LCD_BUCK_MODULE (Autodesk Fusion 360 design; units mm, degrees)
Autodesk Fusion 360 part; units mm, degrees
sketch "Esquisse1" plane through (0, 0, 0) normal (0, 0, 1) x (1, 0, 0)
  line L0 (-36, -19) -> (36, -19)
  line L1 (36, -19) -> (36, 19)
  line L2 (36, 19) -> (-36, 19)
  line L3 (-36, 19) -> (-36, -19)
  line L4 (-36, -19) -> (36, 19) construction
  line L5 (36, -19) -> (-36, 19) construction
  line L6 (-36, -6.0464) -> (-38, -6.0464)
  line L7 (-38, -6.0464) -> (-38, 5.9536)
  line L8 (-38, 5.9536) -> (-36, 5.9536)
  line L9 (-36, 5.9536) -> (-36, -6.0464)
  line L10 (-36, -6.0464) -> (-38, 5.9536) construction
  line L11 (-38, -6.0464) -> (-36, 5.9536) construction
  line L12 (0, 1.75) -> (0, 22.5)
  line L13 (36, -6.0464) -> (38, -6.0464)
  line L14 (36, -6.0464) -> (38, 5.9536) construction
  line L15 (38, -6.0464) -> (36, 5.9536) construction
  line L16 (38, -6.0464) -> (38, 5.9536)
  line L17 (38, 5.9536) -> (36, 5.9536)
  line L18 (36, 5.9536) -> (36, -6.0464)
  point P0 (-37, -0.0464)
  point P1 (37, -0.0464)
  dimension "d1" = 72
  dimension "d2" = 38
  dimension "d3" = 12
  dimension "d4" = 2
  constraint horizontal L0
  constraint perpendicular L0 L1
  constraint parallel L0 L2
  constraint parallel L1 L3
  constraint coincident L4 origin
  constraint coincident L5 origin
  constraint horizontal L6
  constraint perpendicular L6 L7
  constraint parallel L6 L8
  constraint parallel L7 L9
  constraint coincident L10 P0
  constraint coincident L11 P0
  constraint coincident L3 L6.start
  constraint symmetric L6.start L12 L13.start
  constraint symmetric L6.end L12 L13.end
  constraint symmetric L7.end L12 L14.end
  constraint symmetric L8.end L12 L15.end
  constraint symmetric P0 L12 P1
  measures "d1" distance of L1.end L2.end
  measures "d2" distance of L0.start L2.end
  measures "d3" distance of L6.end L7.end
  measures "d4" distance of L6.start L6.end
extrude "Extrusion1" add sketch "Esquisse1" along normal blind 20
sketch "Esquisse2" plane through (0, 0, 0) normal (0, 0, -1) x (1, 0, 0)
  line L0 (-36, 19) -> (-36, 6.0464)
  line L1 (-36, 6.0464) -> (-38, 6.0464)
  line L2 (-38, 6.0464) -> (-38, -5.9536)
  line L3 (-38, -5.9536) -> (-36, -5.9536)
  line L4 (-36, -5.9536) -> (-36, -19)
  line L5 (-36, -19) -> (36, -19)
  line L6 (36, -19) -> (36, -5.9536)
  line L7 (36, -5.9536) -> (38, -5.9536)
  line L8 (38, -5.9536) -> (38, 6.0464)
  line L9 (38, 6.0464) -> (36, 6.0464)
  line L10 (36, 6.0464) -> (36, 19)
  line L11 (36, 19) -> (-36, 19)
  line L12 (30, -15) -> (-30, -15)
  line L13 (-30, -15) -> (-30, 15)
  line L14 (-30, 15) -> (30, 15)
  line L15 (30, 15) -> (30, -15)
  line L16 (30, -15) -> (-30, 15) construction
  line L17 (-30, -15) -> (30, 15) construction
  dimension "d7" = 60
  dimension "d8" = 30
  constraint horizontal L12
  constraint perpendicular L12 L13
  constraint parallel L12 L14
  constraint parallel L13 L15
  constraint coincident L16 origin
  constraint coincident L17 origin
  measures "d7" distance of L13.end L14.end
  measures "d8" distance of L12.end L13.end
extrude "Extrusion2" add sketch "Esquisse2" along normal blind 2 contours L12 L13 L14 L15
